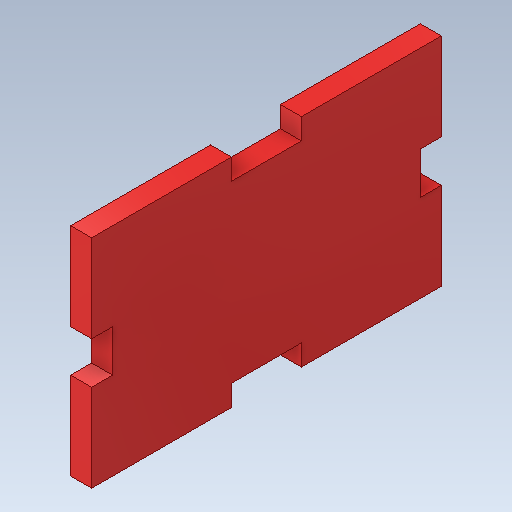
# Autodesk Inventor part: Part7
Saved by Autodesk Inventor 2020 (Build 240168000, 168)
## iProperties
Created: 2020-03-11
Part Number: Part7
Material: Generic
Document SubType Name: Modeling
Designer: tor16003
Density: 1 g/cm^3
Appearance: Light Red
Author: tor16003
Autodesk Inventor part; units mm, degrees
ref_plane "YZ Plane" through (0, 0, 0) normal (1, 0, 0) x (0, 1, 0)
ref_plane "XZ Plane" through (0, 0, 0) normal (0, 1, 0) x (-1, 0, 0)
ref_plane "XY Plane" through (0, 0, 0) normal (0, 0, 1) x (1, 0, 0)
sketch "Sketch1" plane through (0, 0, 0) normal (1, 0, 0) x (0, 1, 0)
  line L0 (0, 0) -> (12.5, 0)
  line L1 (12.5, 0) -> (12.5, -3)
  line L2 (12.5, -3) -> (18.5, -3)
  line L3 (18.5, -3) -> (18.5, 0)
  line L4 (18.5, 0) -> (31, 0)
  line L5 (31, -50) -> (18.5, -50)
  line L6 (18.5, -50) -> (18.5, -47)
  line L7 (18.5, -47) -> (12.5, -47)
  line L8 (12.5, -47) -> (12.5, -50)
  line L9 (12.5, -50) -> (0, -50)
  line L10 (31, 0) -> (31, -20)
  line L11 (31, -20) -> (28, -20)
  line L12 (28, -20) -> (28, -30)
  line L13 (28, -30) -> (31, -30)
  line L14 (31, -30) -> (31, -50)
  line L15 (0, 0) -> (0, -20)
  line L16 (0, -20) -> (3, -20)
  line L17 (3, -20) -> (3, -30)
  line L18 (3, -30) -> (0, -30)
  line L19 (0, -30) -> (0, -50)
  dimension "d2" = 6
  dimension "d14" = 50
  dimension "d16" = 10
  dimension "d19" = 3
  dimension "d22" = 25
  constraints: 40 end point, 13 perpendicular, 9 equal length, 4 vertical, 3 point on line, 2 collinear, 2 horizontal
  measures "d2" distance of L1.end L2.end
  measures "d14" distance between parallel lines of L5 L4
  measures "d16" distance of L16.end L17.end
  measures "d19" distance between parallel lines of L2 L4
  measures "d22" distance between parallel lines of L17 L12
extrude "Extrusion1" add sketch "Sketch1" along normal blind 3
body "Solid1"
